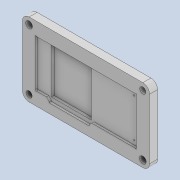
# Autodesk Inventor part: scatola_sotto
Saved by Autodesk Inventor 2022 (Build 260153000, 153)
## iProperties
Created: 2025-09-23
Part Number: scatola_sotto
Material: Generic
Document SubType Name: Modeling
Designer: 1234
Density: 1 g/cm^3
Appearance: Default
Author: 1234
Autodesk Inventor part; units mm, degrees
ref_plane "YZ Plane" through (0, 0, 0) normal (1, 0, 0) x (0, 1, 0)
ref_plane "XZ Plane" through (0, 0, 0) normal (0, 1, 0) x (-1, 0, 0)
ref_plane "XY Plane" through (0, 0, 0) normal (0, 0, 1) x (1, 0, 0)
sketch "Sketch1" plane through (0, 0, 0) normal (0, 0, 1) x (1, 0, 0)
  line L0 (0, 0) -> (-75, 0)
  line L1 (-75, 0) -> (-75, 35)
  line L2 (-75, 35) -> (0, 35)
  line L3 (0, 35) -> (0, 0)
  line L4 (10, -10) -> (-85, -10)
  line L5 (-85, -10) -> (-85, 45)
  line L6 (-85, 45) -> (10, 45)
  line L7 (10, 45) -> (10, -10)
  line L8 (0, 35) -> (10, 45) construction
  circle A0 centre (5, 40) radius 2.25
  arc A1 (10, 40) -> (5, 45) centre (5, 40) ccw
  line L9 (-37.5, 45) -> (-37.5, 54.2273) construction
  circle A2 centre (-80, 40) radius 2.25 construction
  arc A3 (-80, 45) -> (-85, 40) centre (-80, 40) ccw
  line L10 (-85, 17.5) -> (-92.6498, 17.5) construction
  circle A4 centre (5, -5) radius 2.25 construction
  arc A5 (5, -10) -> (10, -5) centre (5, -5) ccw
  circle A6 centre (-80, -5) radius 2.25
  arc A7 (-85, -5) -> (-80, -10) centre (-80, -5) ccw
  line L11 (-65, 0) -> (-65, 35)
  line L12 (-35, 0) -> (-35, 35)
  circle A8 centre (-3, 32) radius 0.5
  circle A9 centre (-3, 3) radius 0.5
  line L13 (-3, 3) -> (-3, 32) construction
  line L14 (-3, 17.5) -> (-10.1857, 17.5) construction
  circle A10 centre (-75, 35) radius 0.5
  circle A11 centre (0, 35) radius 0.5
  circle A12 centre (-75, 0) radius 0.5
  circle A13 centre (0, 0) radius 0.5
  circle A14 centre (-80, 40) radius 2.5
  circle A15 centre (5, -5) radius 2.5
  line L15 (-75.2, 35.2) -> (-75.2, -0.2)
  line L16 (-75.2, -0.2) -> (0.2, -0.2)
  line L17 (0.2, -0.2) -> (0.2, 35.2)
  line L18 (0.2, 35.2) -> (-75.2, 35.2)
  line L19 (-65, 0) -> (-65, -3)
  line L20 (-65, -3) -> (-35, -3)
  line L21 (-35, -3) -> (-35, 0)
  point P0 (5, -10)
  point P1 (-80, 45)
  point P2 (-80, -10)
  point P3 (-0.5, 35)
  point P4 (0, 34.5)
  point P5 (0, 0.5)
  point P6 (-0.5, 0)
  point P7 (-75, 0.5)
  point P8 (-74.5, 0)
  point P9 (-74.5, 35)
  point P10 (-75, 34.5)
  point P11 (0.2, 0.4583)
  point P12 (0.2, 34.5417)
  point P13 (-0.4583, 35.2)
  point P14 (-74.5417, 35.2)
  point P15 (-74.5417, -0.2)
  point P16 (-0.4583, -0.2)
  point P17 (-75.2, 34.5417)
  point P18 (-75.2, 0.4583)
  point P19 (-35, -0.2)
  point P20 (-65, -0.2)
  dimension "d0" = 75
  dimension "d1" = 35
  dimension "d2" = 10
  dimension "d3" = 4.5
  dimension "d8" = 10
  dimension "d9" = 40
  dimension "d10" = 1
  dimension "d11" = 1
  dimension "d12" = 29
  dimension "d13" = 3
  dimension "d18" = 1
  dimension "d21" = 75
  dimension "d24" = 35
  dimension "d30" = 5
  dimension "d31" = 5
  dimension "d32" = 0.2
  dimension "d33" = 3
  constraints: 44 end point, 16 centre point, 12 symmetric about line, 9 perpendicular, 8 point on circle, 7 coincident, 6 parallel, 6 point on line, 4 midpoint, 3 horizontal, 3 vertical, 1 collinear, 1 tangent, 18 other
  measures "d0" distance of L1.end L2.end
  measures "d1" distance of L0.end L1.end
  measures "d2" distance between parallel lines of L3 L7
  measures "d3" diameter of A0
  measures "d8" distance between parallel lines of L1 L11
  measures "d9" distance between parallel lines of L1 L12
  measures "d10" diameter of A9
  measures "d11" diameter of A8
  measures "d12" distance of L13.start L13.end
  measures "d13" distance between parallel lines of L3 L13
  measures "d18" diameter of A10
  measures "d21" distance of A10.centre A11.centre
  measures "d24" distance of A10.centre A12.centre
  measures "d30" diameter of A14
  measures "d31" diameter of A15
  measures "d32" distance between parallel lines of L1 L15
  measures "d33" distance between parallel lines of L0 L20
extrude "Extrusion1" add sketch "Sketch1" along normal blind 6 contours L21 L16 L19 L0 | L12 L2 A11 L3 A13 L0 | L0 L11 L2 L12 | L0 A13 L16 L21 | L19 L16 A12 L0 | L0 A12 L1 A10 L2 L11 | A13 L3 L0 | L0 L3 A13 L17 L16 | L2 A10 L18 A11 | L21 L20 L19 L16 | A12 L16 L15 L1 L0 | L0 L1 A12 | L3 A11 L17 A13 | L16 L17 A13 | A11 L18 L17 L3 L2 | L2 L3 A11 | A12 L15 A10 L1 | A12 L15 L16 | A10 L1 L2 | L2 L1 A10 L15 L18 | A11 L17 L18 | L18 L15 A10 | L4 A7 L5 A3 L6 A1 L7 A5 | A8 | A9
extrude "Extrusion2" cut sketch "Sketch1" against normal blind 1.6 from surface at 6 contours L21 L16 L19 L0 | L12 L2 A11 L3 A13 L0 | L0 L11 L2 L12 | L0 A13 L16 L21 | L19 L16 A12 L0 | L0 A12 L1 A10 L2 L11 | A13 L3 L0 | L0 L3 A13 L17 L16 | L2 A10 L18 A11 | L21 L20 L19 L16 | A12 L16 L15 L1 L0 | L0 L1 A12 | L3 A11 L17 A13 | L16 L17 A13 | A11 L18 L17 L3 L2 | L2 L3 A11 | A12 L15 A10 L1 | A12 L15 L16 | A10 L1 L2 | L2 L1 A10 L15 L18 | A11 L17 L18 | L18 L15 A10 | A8 | A9
extrude "Extrusion3" cut sketch "Sketch1" against normal blind 2 from surface at 4.4 contours L0 L11 L2 L12
extrude "Extrusion4" cut sketch "Sketch1" against normal blind 3 from surface at 4.4 contours A8 | A9
chamfer "Chamfer2" distance 2 angle 45 2 edges at (-65, -0.2, 5.2) (-35, -0.2, 5.2)
equation "\"d11\" = d10"
equation "\"d21\" = d0"
equation "\"d24\" = d1"
equation "\"d31\" = d30"
body "Solid1"
